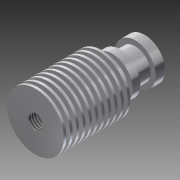
# Autodesk Inventor part: e3d_v6_heatsink
Saved by Autodesk Inventor 2013 (Build 170138000, 138)
## iProperties
Created: 2015-02-20
Part Number: e3d_v6_heatsink
Material: 一般
Document SubType Name: Modeling
Designer: Noa Izumi
Density: 1 g/cm^3
Author: Noa Izumi
Autodesk Inventor part; units mm, degrees
ref_plane "YZ Plane" through (0, 0, 0) normal (1, 0, 0) x (0, 1, 0)
ref_plane "XZ Plane" through (0, 0, 0) normal (0, 1, 0) x (-1, 0, 0)
ref_plane "XY Plane" through (0, 0, 0) normal (0, 0, 1) x (1, 0, 0)
sketch "草圖1" plane through (0, 0, 0) normal (0, 0, 1) x (1, 0, 0)
  line L0 (0, 0) -> (-11.15, 0)
  line L1 (-11.15, 0) -> (-11.15, 1)
  line L2 (-11.15, 1) -> (0, 1)
  line L3 (0, 1) -> (0, 0)
  line L4 (0, 2.5) -> (-11.15, 2.5)
  line L5 (-11.15, 2.5) -> (-11.15, 3.5)
  line L6 (-11.15, 3.5) -> (0, 3.5)
  line L7 (0, 3.5) -> (0, 2.5)
  line L8 (0, 5) -> (-11.15, 5)
  line L9 (-11.15, 5) -> (-11.15, 6)
  line L10 (-11.15, 6) -> (0, 6)
  line L11 (0, 6) -> (0, 5)
  line L12 (0, 7.5) -> (-11.15, 7.5)
  line L13 (-11.15, 7.5) -> (-11.15, 8.5)
  line L14 (-11.15, 8.5) -> (0, 8.5)
  line L15 (0, 8.5) -> (0, 7.5)
  line L16 (0, 10) -> (-11.15, 10)
  line L17 (-11.15, 10) -> (-11.15, 11)
  line L18 (-11.15, 11) -> (0, 11)
  line L19 (0, 11) -> (0, 10)
  line L20 (0, 12.5) -> (-11.15, 12.5)
  line L21 (-11.15, 12.5) -> (-11.15, 13.5)
  line L22 (-11.15, 13.5) -> (0, 13.5)
  line L23 (0, 13.5) -> (0, 12.5)
  line L24 (0, 15) -> (-11.15, 15)
  line L25 (-11.15, 15) -> (-11.15, 16)
  line L26 (-11.15, 16) -> (0, 16)
  line L27 (0, 16) -> (0, 15)
  line L28 (0, 17.5) -> (-11.15, 17.5)
  line L29 (-11.15, 17.5) -> (-11.15, 18.5)
  line L30 (-11.15, 18.5) -> (0, 18.5)
  line L31 (0, 18.5) -> (0, 17.5)
  line L32 (0, 20) -> (-11.15, 20)
  line L33 (-11.15, 20) -> (-11.15, 21)
  line L34 (-11.15, 21) -> (0, 21)
  line L35 (0, 21) -> (0, 20)
  line L36 (0, 22.5) -> (-11.15, 22.5)
  line L37 (-11.15, 22.5) -> (-11.15, 23.5)
  line L38 (-11.15, 23.5) -> (0, 23.5)
  line L39 (0, 23.5) -> (0, 22.5)
  line L40 (0, 25) -> (-11.15, 25)
  line L41 (-11.15, 25) -> (-11.15, 26)
  line L42 (-11.15, 26) -> (0, 26)
  line L43 (0, 26) -> (0, 25)
  line L44 (-5.65, 0) -> (-4.5, 26)
  line L45 (-4.5, 26) -> (0, 26)
  line L46 (0, 0) -> (-5.65, 0)
  line L47 (0, 26) -> (0, 0)
  line L48 (0, 42.7) -> (-8, 42.7)
  line L49 (-8, 42.7) -> (-8, 39)
  line L50 (-8, 39) -> (0, 39)
  line L51 (0, 39) -> (0, 42.7)
  line L52 (-8, 33) -> (0, 33)
  line L53 (0, 33) -> (0, 30)
  line L54 (0, 30) -> (-8, 30)
  line L55 (-8, 30) -> (-8, 33)
  line L56 (-6, 39) -> (0, 39)
  line L57 (0, 39) -> (0, 33)
  line L58 (0, 33) -> (-6, 33)
  line L59 (-6, 33) -> (-6, 39)
  line L60 (-8, 28.5) -> (0, 28.5)
  line L61 (0, 28.5) -> (0, 27.5)
  line L62 (0, 27.5) -> (-8, 27.5)
  line L63 (-8, 27.5) -> (-8, 28.5)
  line L64 (-4.5, 26) -> (0, 26)
  line L65 (0, 26) -> (0, 30)
  line L66 (0, 30) -> (-4.5, 30)
  line L67 (-4.5, 30) -> (-4.5, 26)
  dimension "d2" = 11.15
  dimension "d3" = 1
  dimension "d9" = 2.5
  dimension "d11" = 5.5
  dimension "d12" = 4.5
  dimension "d14" = 42.7
  dimension "d15" = 3.7
  dimension "d16" = 3
  dimension "d17" = 8
  dimension "d19" = 6
  dimension "d20" = 6
  dimension "d21" = 1
  dimension "d22" = 1.5
  constraints: 136 end point, 13 parallel, 7 perpendicular, 6 horizontal, 4 point on line, 2 collinear, 1 vertical, 79 other
  measures "d2" distance of L0.start L0.end
  measures "d3" distance of L0.end L1.end
  measures "d9" distance of L0.start L4.start
  measures "d11" distance from line of L44.start L1
  measures "d12" distance from line of L43 L44.end
  measures "d14" distance between parallel lines of L0 L48
  measures "d15" distance of L50.end L48.start
  measures "d16" distance of L52.end L53.end
  measures "d17" distance of L48.start L48.end
  measures "d19" distance between parallel lines of L52 L50
  measures "d20" distance between parallel lines of L57 L59
  measures "d21" distance of L60.end L61.end
  measures "d22" distance between parallel lines of L42 L62
revolve "迴轉1" add sketch "草圖1" angle 360 about axis through (0, 26, 0) along (0, -1, 0)
sketch "草圖2" plane through (0, 0, 0) normal (0, -1, 0) x (1, 0, 0)
  circle A0 centre (0, 0) radius 11.15 projected
  constraints: 1 coincident
hole "孔1" at (0, 0, 0) direction (0, 1, 0) diameter 5.917 depth 14.8 tip angle 118 thread size "M7x1" class "6H" standard "ANSI Metric M Profile"
sketch "草圖3" plane through (0, 42.7, 0) normal (0, 1, 0) x (1, 0, 0)
  circle A0 centre (0, 0) radius 8 projected
  constraints: 1 coincident
hole "孔2" at (0, 42.7, 0) direction (0, -1, 0) diameter 2 end through all
sketch "草圖4" plane through (0, 42.7, 0) normal (0, 1, 0) x (1, 0, 0)
  circle A0 centre (0, 0) radius 8 projected
  constraints: 1 coincident
hole "孔3" at (0, 42.7, 0) direction (0, -1, 0) diameter 8.376 depth 6 tip angle 118 thread size "M10x1.5" class "6H" standard "ANSI Metric M Profile"
